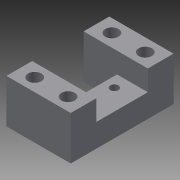
# Autodesk Inventor part: servo_clip_holder1_final
Saved by Autodesk Inventor 2015 (Build 190159000, 159)
## iProperties
Created: 2018-01-08
Part Number: servo_clip_holder1_final
Material: Generic
Document SubType Name: Modeling
Designer: Anshul
Density: 1 g/cm^3
Appearance: Default
Author: Anshul
Autodesk Inventor part; units mm, degrees
ref_plane "YZ Plane" through (0, 0, 0) normal (1, 0, 0) x (0, 1, 0)
ref_plane "XZ Plane" through (0, 0, 0) normal (0, 1, 0) x (-1, 0, 0)
ref_plane "XY Plane" through (0, 0, 0) normal (0, 0, 1) x (1, 0, 0)
sketch "Sketch1" plane through (0, 0, 0) normal (0, 1, 0) x (-1, 0, 0)
  line L0 (0, 0) -> (0, -10)
  line L1 (0, 0) -> (0, 10)
  line L2 (0, 10) -> (13, 10)
  line L3 (13, 10) -> (13, 20)
  line L4 (13, 20) -> (-12, 20)
  line L5 (0, -10) -> (13, -10)
  line L6 (13, -10) -> (13, -20)
  line L7 (13, -20) -> (-12, -20)
  line L8 (-12, -20) -> (-12, 20)
  line L9 (-12, 15) -> (-6, 15)
  line L10 (13, 15) -> (7, 15)
  line L11 (13, -15) -> (7, -15)
  line L12 (-12, -15) -> (-6, -15)
  circle A0 centre (7, 15) radius 2.6
  circle A1 centre (-6, 15) radius 2.6
  circle A2 centre (-6, -15) radius 2.6
  circle A3 centre (7, -15) radius 2.6
  line L13 (0, 0) -> (-4, 0)
  line L14 (-4, 0) -> (-4, -5)
  line L15 (-4, 0) -> (-4, 5)
  circle A4 centre (-4, 5) radius 1.6
  circle A5 centre (-4, -5) radius 1.6
  line L16 (0, 10) -> (-12, 10)
  line L17 (0, -10) -> (-12, -10)
  line L18 (13, -15) -> (9.6, -15)
  line L19 (-8.6, -15) -> (-12, -15)
  line L20 (13, 15) -> (9.6, 15)
  line L21 (-8.6, 15) -> (-12, 15)
  dimension "d12" = 5.2
  dimension "d13" = 5.2
  dimension "d14" = 5.2
  dimension "d15" = 5.2
  dimension "d0" = 10
  dimension "d1" = 10
  dimension "d2" = 13
  dimension "d3" = 10
  dimension "d4" = 25
  dimension "d5" = 13
  dimension "d6" = 10
  dimension "d7" = 25
  dimension "d8" = 6
  dimension "d9" = 6
  dimension "d10" = 6
  dimension "d11" = 6
  dimension "d16" = 4
  dimension "d17" = 5
  dimension "d18" = 5
  dimension "d19" = 3.2
  dimension "d20" = 3.2
  constraints: 44 end point, 12 point on line, 10 perpendicular, 6 coincident, 4 horizontal alignment, 2 centre point, 2 midpoint, 2 vertical, 1 horizontal, 8 other
  measures "d0" distance of L0.start L0.end
  measures "d1" distance of L0.start L1.end
  measures "d2" distance of L1.end L2.end
  measures "d3" distance of L2.end L3.end
  measures "d4" distance of L3.end L4.end
  measures "d5" distance of L0.end L5.end
  measures "d6" distance of L5.end L6.end
  measures "d7" distance of L6.end L7.end
  measures "d8" distance of L9.start L9.end
  measures "d9" distance of L10.start L10.end
  measures "d10" distance of L11.start L11.end
  measures "d11" distance of L12.start L12.end
  measures "d16" distance of L0.start L13.end
  measures "d17" distance of L13.end L14.end
  measures "d18" distance of L13.end L15.end
  measures "d19" diameter of A4
  measures "d20" diameter of A5
extrude "Extrusion1" add sketch "Sketch1" along normal blind 17 contours L5 L6 L7 L8 L17 | L16 L8 L4 L3 L2
extrude "Extrusion2" add sketch "Sketch1" along normal blind 9 contours L0 L17 L8 L16 L1
body "Solid1"
